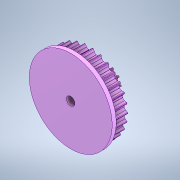
# Autodesk Inventor part: TransmissionCenterBigPulley HTD3M
Saved by Autodesk Inventor 2022.2 (Build 262287000, 287)
## iProperties
CustomPartVersion: 1
Created: 2022-01-04
Part Number: TransmissionCenterBigPulley HTD3M
Material: Steel
Document SubType Name: Modeling
Designer: Jochen
Density: 1 g/cm^3
Appearance: Steel
Author: Jochen
Autodesk Inventor part; units mm, degrees
ref_plane "YZ Plane" through (0, 0, 0) normal (1, 0, 0) x (0, 1, 0)
ref_plane "XZ Plane" through (0, 0, 0) normal (0, 1, 0) x (-1, 0, 0)
ref_plane "XY Plane" through (0, 0, 0) normal (0, 0, 1) x (1, 0, 0)
sketch "Pulley" plane through (0, 0, 0) normal (0, 0, 1) x (1, 0, 0)
  line L0 (0, -20.7693) -> (0, 20.7693) construction
  line L1 (-20.7693, 0) -> (20.7693, 0) construction
  circle A0 centre (0, 0) radius 14
  circle A1 centre (0, 0) radius 1.5
  arc A2 (-1.5293, 13.8609) -> (-1.6879, 13.7364) centre (-1.5084, 13.671) ccw
  arc A3 (-1.3859, 13.876) -> (-1.5293, 13.8609) centre (0, 0) ccw
  arc A4 (-1.205, 13.7871) -> (-1.3859, 13.876) centre (-1.3669, 13.6859) ccw
  line L2 (-1.205, 13.7871) -> (-0.8141, 13.1617)
  arc A5 (-0.8141, 13.1617) -> (-0.028, 12.726) centre (-0.028, 13.653) ccw
  line L3 (-0.028, 12.726) -> (0.028, 12.726)
  arc A6 (0.028, 12.726) -> (0.8141, 13.1617) centre (0.028, 13.653) ccw
  line L4 (0.8141, 13.1617) -> (1.205, 13.7871)
  arc A7 (1.3859, 13.876) -> (1.205, 13.7871) centre (1.3669, 13.6859) ccw
  arc A8 (1.5293, 13.8609) -> (1.3859, 13.876) centre (0, 0) ccw
  arc A9 (1.6879, 13.7364) -> (1.5293, 13.8609) centre (1.5084, 13.671) ccw
  line L5 (1.6879, 13.7364) -> (1.9402, 13.0434)
  arc A10 (1.9402, 13.0434) -> (2.6185, 12.4537) centre (2.8112, 13.3605) ccw
  line L6 (2.6185, 12.4537) -> (2.6733, 12.4421)
  arc A11 (2.6733, 12.4421) -> (3.5328, 12.7048) centre (2.866, 13.3488) ccw
  line L7 (3.5328, 12.7048) -> (4.0451, 13.2353)
  arc A12 (4.2406, 13.2846) -> (4.0451, 13.2353) centre (4.1825, 13.1026) ccw
  arc A13 (4.3778, 13.24) -> (4.2406, 13.2846) centre (0, 0) ccw
  arc A14 (4.5069, 13.0853) -> (4.3778, 13.24) centre (4.3178, 13.0587) ccw
  line L8 (4.5069, 13.0853) -> (4.6096, 12.3549)
  arc A15 (4.6096, 12.3549) -> (5.1506, 11.6372) centre (5.5276, 12.484) ccw
  line L9 (5.1506, 11.6372) -> (5.2017, 11.6144)
  arc A16 (5.2017, 11.6144) -> (6.0971, 11.6927) centre (5.5788, 12.4612) ccw
  line L10 (6.0971, 11.6927) -> (6.7085, 12.1051)
  arc A17 (6.91, 12.1126) -> (6.7085, 12.1051) centre (6.8153, 11.9467) ccw
  arc A18 (7.0348, 12.0405) -> (6.91, 12.1126) centre (0, 0) ccw
  arc A19 (7.129, 11.8623) -> (7.0348, 12.0405) centre (6.9385, 11.8756) ccw
  line L11 (7.129, 11.8623) -> (7.0776, 11.1266)
  arc A20 (7.0776, 11.1266) -> (7.4575, 10.312) centre (8.0024, 11.062) ccw
  line L12 (7.4575, 10.312) -> (7.5028, 10.2791)
  arc A21 (7.5028, 10.2791) -> (8.3949, 10.1695) centre (8.0477, 11.0291) ccw
  line L13 (8.3949, 10.1695) -> (9.0787, 10.4458)
  arc A22 (9.2773, 10.4113) -> (9.0787, 10.4458) centre (9.1503, 10.2687) ccw
  arc A23 (9.3845, 10.3148) -> (9.2773, 10.4113) centre (0, 0) ccw
  arc A24 (9.4395, 10.1209) -> (9.3845, 10.3148) centre (9.2559, 10.1735) ccw
  line L14 (9.4395, 10.1209) -> (9.2363, 9.4119)
  arc A25 (9.2363, 9.4119) -> (9.4385, 8.5362) centre (10.1274, 9.1564) ccw
  line L15 (9.4385, 8.5362) -> (9.476, 8.4945)
  arc A26 (9.476, 8.4945) -> (10.3258, 8.2019) centre (10.1649, 9.1148) ccw
  line L16 (10.3258, 8.2019) -> (11.0521, 8.3299)
  arc A27 (11.2392, 8.2549) -> (11.0521, 8.3299) centre (11.0853, 8.1418) ccw
  arc A28 (11.324, 8.1382) -> (11.2392, 8.2549) centre (0, 0) ccw
  arc A29 (11.3375, 7.9371) -> (11.324, 8.1382) centre (11.1689, 8.0268) ccw
  line L17 (11.3375, 7.9371) -> (10.9913, 7.2859)
  arc A30 (10.9913, 7.2859) -> (11.007, 6.3872) centre (11.8098, 6.8507) ccw
  line L18 (11.007, 6.3872) -> (11.035, 6.3388)
  arc A31 (11.035, 6.3388) -> (11.8054, 5.8758) centre (11.8378, 6.8023) ccw
  line L19 (11.8054, 5.8758) -> (12.5425, 5.85)
  arc A32 (12.7099, 5.7377) -> (12.5425, 5.85) centre (12.5358, 5.6591) ccw
  arc A33 (12.7685, 5.606) -> (12.7099, 5.7377) centre (0, 0) ccw
  arc A34 (12.74, 5.4065) -> (12.7685, 5.606) centre (12.5937, 5.5292) ccw
  line L20 (12.74, 5.4065) -> (12.266, 4.8415)
  arc A35 (12.266, 4.8415) -> (12.0945, 3.9592) centre (12.9761, 4.2456) ccw
  line L21 (12.0945, 3.9592) -> (12.1118, 3.9059)
  arc A36 (12.1118, 3.9059) -> (12.7691, 3.2929) centre (12.9934, 4.1924) ccw
  line L22 (12.7691, 3.2929) -> (13.4847, 3.1145)
  arc A37 (13.6251, 2.9698) -> (13.4847, 3.1145) centre (13.4385, 2.9291) ccw
  arc A38 (13.6551, 2.8288) -> (13.6251, 2.9698) centre (0, 0) ccw
  arc A39 (13.5856, 2.6395) -> (13.6551, 2.8288) centre (13.468, 2.79) ccw
  line L23 (13.5856, 2.6395) -> (13.0045, 2.1854)
  arc A40 (13.0045, 2.1854) -> (12.6534, 1.3581) centre (13.5753, 1.455) ccw
  line L24 (12.6534, 1.3581) -> (12.6592, 1.3024)
  arc A41 (12.6592, 1.3024) -> (13.1747, 0.5661) centre (13.5811, 1.3993) ccw
  line L25 (13.1747, 0.5661) -> (13.8376, 0.2428)
  arc A42 (13.9448, 0.0721) -> (13.8376, 0.2428) centre (13.7538, 0.0711) ccw
  arc A43 (13.9448, -0.0721) -> (13.9448, 0.0721) centre (0, 0) ccw
  arc A44 (13.8376, -0.2428) -> (13.9448, -0.0721) centre (13.7538, -0.0711) ccw
  line L26 (13.8376, -0.2428) -> (13.1747, -0.5661)
  arc A45 (13.1747, -0.5661) -> (12.6592, -1.3024) centre (13.5811, -1.3993) ccw
  line L27 (12.6592, -1.3024) -> (12.6534, -1.3581)
  arc A46 (12.6534, -1.3581) -> (13.0045, -2.1854) centre (13.5753, -1.455) ccw
  line L28 (13.0045, -2.1854) -> (13.5856, -2.6395)
  arc A47 (13.6551, -2.8288) -> (13.5856, -2.6395) centre (13.468, -2.79) ccw
  arc A48 (13.6251, -2.9698) -> (13.6551, -2.8288) centre (0, 0) ccw
  arc A49 (13.4847, -3.1145) -> (13.6251, -2.9698) centre (13.4385, -2.9291) ccw
  line L29 (13.4847, -3.1145) -> (12.7691, -3.2929)
  arc A50 (12.7691, -3.2929) -> (12.1118, -3.9059) centre (12.9934, -4.1924) ccw
  line L30 (12.1118, -3.9059) -> (12.0945, -3.9592)
  arc A51 (12.0945, -3.9592) -> (12.266, -4.8415) centre (12.9761, -4.2456) ccw
  line L31 (12.266, -4.8415) -> (12.74, -5.4065)
  arc A52 (12.7685, -5.606) -> (12.74, -5.4065) centre (12.5937, -5.5292) ccw
  arc A53 (12.7099, -5.7377) -> (12.7685, -5.606) centre (0, 0) ccw
  arc A54 (12.5425, -5.85) -> (12.7099, -5.7377) centre (12.5358, -5.6591) ccw
  line L32 (12.5425, -5.85) -> (11.8054, -5.8758)
  arc A55 (11.8054, -5.8758) -> (11.035, -6.3388) centre (11.8378, -6.8023) ccw
  line L33 (11.035, -6.3388) -> (11.007, -6.3872)
  arc A56 (11.007, -6.3872) -> (10.9913, -7.2859) centre (11.8098, -6.8507) ccw
  line L34 (10.9913, -7.2859) -> (11.3375, -7.9371)
  arc A57 (11.324, -8.1382) -> (11.3375, -7.9371) centre (11.1689, -8.0268) ccw
  arc A58 (11.2392, -8.2549) -> (11.324, -8.1382) centre (0, 0) ccw
  arc A59 (11.0521, -8.3299) -> (11.2392, -8.2549) centre (11.0853, -8.1418) ccw
  line L35 (11.0521, -8.3299) -> (10.3258, -8.2019)
  arc A60 (10.3258, -8.2019) -> (9.476, -8.4945) centre (10.1649, -9.1148) ccw
  line L36 (9.476, -8.4945) -> (9.4385, -8.5362)
  arc A61 (9.4385, -8.5362) -> (9.2363, -9.4119) centre (10.1274, -9.1564) ccw
  line L37 (9.2363, -9.4119) -> (9.4395, -10.1209)
  arc A62 (9.3845, -10.3148) -> (9.4395, -10.1209) centre (9.2559, -10.1735) ccw
  arc A63 (9.2773, -10.4113) -> (9.3845, -10.3148) centre (0, 0) ccw
  arc A64 (9.0787, -10.4458) -> (9.2773, -10.4113) centre (9.1503, -10.2687) ccw
  line L38 (9.0787, -10.4458) -> (8.3949, -10.1695)
  arc A65 (8.3949, -10.1695) -> (7.5028, -10.2791) centre (8.0477, -11.0291) ccw
  line L39 (7.5028, -10.2791) -> (7.4575, -10.312)
  arc A66 (7.4575, -10.312) -> (7.0776, -11.1266) centre (8.0024, -11.062) ccw
  line L40 (7.0776, -11.1266) -> (7.129, -11.8623)
  arc A67 (7.0348, -12.0405) -> (7.129, -11.8623) centre (6.9385, -11.8756) ccw
  arc A68 (6.91, -12.1126) -> (7.0348, -12.0405) centre (0, 0) ccw
  arc A69 (6.7085, -12.1051) -> (6.91, -12.1126) centre (6.8153, -11.9467) ccw
  line L41 (6.7085, -12.1051) -> (6.0971, -11.6927)
  arc A70 (6.0971, -11.6927) -> (5.2017, -11.6144) centre (5.5788, -12.4612) ccw
  line L42 (5.2017, -11.6144) -> (5.1506, -11.6372)
  arc A71 (5.1506, -11.6372) -> (4.6096, -12.3549) centre (5.5276, -12.484) ccw
  line L43 (4.6096, -12.3549) -> (4.5069, -13.0853)
  arc A72 (4.3778, -13.24) -> (4.5069, -13.0853) centre (4.3178, -13.0587) ccw
  arc A73 (4.2406, -13.2846) -> (4.3778, -13.24) centre (0, 0) ccw
  arc A74 (4.0451, -13.2353) -> (4.2406, -13.2846) centre (4.1825, -13.1026) ccw
  line L44 (4.0451, -13.2353) -> (3.5328, -12.7048)
  arc A75 (3.5328, -12.7048) -> (2.6733, -12.4421) centre (2.866, -13.3488) ccw
  line L45 (2.6733, -12.4421) -> (2.6185, -12.4537)
  arc A76 (2.6185, -12.4537) -> (1.9402, -13.0434) centre (2.8112, -13.3605) ccw
  line L46 (1.9402, -13.0434) -> (1.6879, -13.7364)
  arc A77 (1.5293, -13.8609) -> (1.6879, -13.7364) centre (1.5084, -13.671) ccw
  arc A78 (1.3859, -13.876) -> (1.5293, -13.8609) centre (0, 0) ccw
  arc A79 (1.205, -13.7871) -> (1.3859, -13.876) centre (1.3669, -13.6859) ccw
  line L47 (1.205, -13.7871) -> (0.8141, -13.1617)
  arc A80 (0.8141, -13.1617) -> (0.028, -12.726) centre (0.028, -13.653) ccw
  line L48 (0.028, -12.726) -> (-0.028, -12.726)
  arc A81 (-0.028, -12.726) -> (-0.8141, -13.1617) centre (-0.028, -13.653) ccw
  line L49 (-0.8141, -13.1617) -> (-1.205, -13.7871)
  arc A82 (-1.3859, -13.876) -> (-1.205, -13.7871) centre (-1.3669, -13.6859) ccw
  arc A83 (-1.5293, -13.8609) -> (-1.3859, -13.876) centre (0, 0) ccw
  arc A84 (-1.6879, -13.7364) -> (-1.5293, -13.8609) centre (-1.5084, -13.671) ccw
  line L50 (-1.6879, -13.7364) -> (-1.9402, -13.0434)
  arc A85 (-1.9402, -13.0434) -> (-2.6185, -12.4537) centre (-2.8112, -13.3605) ccw
  line L51 (-2.6185, -12.4537) -> (-2.6733, -12.4421)
  arc A86 (-2.6733, -12.4421) -> (-3.5328, -12.7048) centre (-2.866, -13.3488) ccw
  line L52 (-3.5328, -12.7048) -> (-4.0451, -13.2353)
  arc A87 (-4.2406, -13.2846) -> (-4.0451, -13.2353) centre (-4.1825, -13.1026) ccw
  arc A88 (-4.3778, -13.24) -> (-4.2406, -13.2846) centre (0, 0) ccw
  arc A89 (-4.5069, -13.0853) -> (-4.3778, -13.24) centre (-4.3178, -13.0587) ccw
  line L53 (-4.5069, -13.0853) -> (-4.6096, -12.3549)
  arc A90 (-4.6096, -12.3549) -> (-5.1506, -11.6372) centre (-5.5276, -12.484) ccw
  line L54 (-5.1506, -11.6372) -> (-5.2017, -11.6144)
  arc A91 (-5.2017, -11.6144) -> (-6.0971, -11.6927) centre (-5.5788, -12.4612) ccw
  line L55 (-6.0971, -11.6927) -> (-6.7085, -12.1051)
  arc A92 (-6.91, -12.1126) -> (-6.7085, -12.1051) centre (-6.8153, -11.9467) ccw
  arc A93 (-7.0348, -12.0405) -> (-6.91, -12.1126) centre (0, 0) ccw
  arc A94 (-7.129, -11.8623) -> (-7.0348, -12.0405) centre (-6.9385, -11.8756) ccw
  line L56 (-7.129, -11.8623) -> (-7.0776, -11.1266)
  arc A95 (-7.0776, -11.1266) -> (-7.4575, -10.312) centre (-8.0024, -11.062) ccw
  line L57 (-7.4575, -10.312) -> (-7.5028, -10.2791)
  arc A96 (-7.5028, -10.2791) -> (-8.3949, -10.1695) centre (-8.0477, -11.0291) ccw
  line L58 (-8.3949, -10.1695) -> (-9.0787, -10.4458)
  arc A97 (-9.2773, -10.4113) -> (-9.0787, -10.4458) centre (-9.1503, -10.2687) ccw
  arc A98 (-9.3845, -10.3148) -> (-9.2773, -10.4113) centre (0, 0) ccw
  arc A99 (-9.4395, -10.1209) -> (-9.3845, -10.3148) centre (-9.2559, -10.1735) ccw
  line L59 (-9.4395, -10.1209) -> (-9.2363, -9.4119)
  arc A100 (-9.2363, -9.4119) -> (-9.4385, -8.5362) centre (-10.1274, -9.1564) ccw
  line L60 (-9.4385, -8.5362) -> (-9.476, -8.4945)
  arc A101 (-9.476, -8.4945) -> (-10.3258, -8.2019) centre (-10.1649, -9.1148) ccw
  line L61 (-10.3258, -8.2019) -> (-11.0521, -8.3299)
  arc A102 (-11.2392, -8.2549) -> (-11.0521, -8.3299) centre (-11.0853, -8.1418) ccw
  arc A103 (-11.324, -8.1382) -> (-11.2392, -8.2549) centre (0, 0) ccw
  arc A104 (-11.3375, -7.9371) -> (-11.324, -8.1382) centre (-11.1689, -8.0268) ccw
  line L62 (-11.3375, -7.9371) -> (-10.9913, -7.2859)
  arc A105 (-10.9913, -7.2859) -> (-11.007, -6.3872) centre (-11.8098, -6.8507) ccw
  line L63 (-11.007, -6.3872) -> (-11.035, -6.3388)
  arc A106 (-11.035, -6.3388) -> (-11.8054, -5.8758) centre (-11.8378, -6.8023) ccw
  line L64 (-11.8054, -5.8758) -> (-12.5425, -5.85)
  arc A107 (-12.7099, -5.7377) -> (-12.5425, -5.85) centre (-12.5358, -5.6591) ccw
  arc A108 (-12.7685, -5.606) -> (-12.7099, -5.7377) centre (0, 0) ccw
  arc A109 (-12.74, -5.4065) -> (-12.7685, -5.606) centre (-12.5937, -5.5292) ccw
  line L65 (-12.74, -5.4065) -> (-12.266, -4.8415)
  arc A110 (-12.266, -4.8415) -> (-12.0945, -3.9592) centre (-12.9761, -4.2456) ccw
  line L66 (-12.0945, -3.9592) -> (-12.1118, -3.9059)
  arc A111 (-12.1118, -3.9059) -> (-12.7691, -3.2929) centre (-12.9934, -4.1924) ccw
  line L67 (-12.7691, -3.2929) -> (-13.4847, -3.1145)
  arc A112 (-13.6251, -2.9698) -> (-13.4847, -3.1145) centre (-13.4385, -2.9291) ccw
  arc A113 (-13.6551, -2.8288) -> (-13.6251, -2.9698) centre (0, 0) ccw
  arc A114 (-13.5856, -2.6395) -> (-13.6551, -2.8288) centre (-13.468, -2.79) ccw
  line L68 (-13.5856, -2.6395) -> (-13.0045, -2.1854)
  arc A115 (-13.0045, -2.1854) -> (-12.6534, -1.3581) centre (-13.5753, -1.455) ccw
  line L69 (-12.6534, -1.3581) -> (-12.6592, -1.3024)
  arc A116 (-12.6592, -1.3024) -> (-13.1747, -0.5661) centre (-13.5811, -1.3993) ccw
  line L70 (-13.1747, -0.5661) -> (-13.8376, -0.2428)
  arc A117 (-13.9448, -0.0721) -> (-13.8376, -0.2428) centre (-13.7538, -0.0711) ccw
  arc A118 (-13.9448, 0.0721) -> (-13.9448, -0.0721) centre (0, 0) ccw
  arc A119 (-13.8376, 0.2428) -> (-13.9448, 0.0721) centre (-13.7538, 0.0711) ccw
  line L71 (-13.8376, 0.2428) -> (-13.1747, 0.5661)
  arc A120 (-13.1747, 0.5661) -> (-12.6592, 1.3024) centre (-13.5811, 1.3993) ccw
  line L72 (-12.6592, 1.3024) -> (-12.6534, 1.3581)
  arc A121 (-12.6534, 1.3581) -> (-13.0045, 2.1854) centre (-13.5753, 1.455) ccw
  line L73 (-13.0045, 2.1854) -> (-13.5856, 2.6395)
  arc A122 (-13.6551, 2.8288) -> (-13.5856, 2.6395) centre (-13.468, 2.79) ccw
  arc A123 (-13.6251, 2.9698) -> (-13.6551, 2.8288) centre (0, 0) ccw
  arc A124 (-13.4847, 3.1145) -> (-13.6251, 2.9698) centre (-13.4385, 2.9291) ccw
  line L74 (-13.4847, 3.1145) -> (-12.7691, 3.2929)
  arc A125 (-12.7691, 3.2929) -> (-12.1118, 3.9059) centre (-12.9934, 4.1924) ccw
  line L75 (-12.1118, 3.9059) -> (-12.0945, 3.9592)
  arc A126 (-12.0945, 3.9592) -> (-12.266, 4.8415) centre (-12.9761, 4.2456) ccw
  line L76 (-12.266, 4.8415) -> (-12.74, 5.4065)
  arc A127 (-12.7685, 5.606) -> (-12.74, 5.4065) centre (-12.5937, 5.5292) ccw
  arc A128 (-12.7099, 5.7377) -> (-12.7685, 5.606) centre (0, 0) ccw
  arc A129 (-12.5425, 5.85) -> (-12.7099, 5.7377) centre (-12.5358, 5.6591) ccw
  line L77 (-12.5425, 5.85) -> (-11.8054, 5.8758)
  arc A130 (-11.8054, 5.8758) -> (-11.035, 6.3388) centre (-11.8378, 6.8023) ccw
  line L78 (-11.035, 6.3388) -> (-11.007, 6.3872)
  arc A131 (-11.007, 6.3872) -> (-10.9913, 7.2859) centre (-11.8098, 6.8507) ccw
  line L79 (-10.9913, 7.2859) -> (-11.3375, 7.9371)
  arc A132 (-11.324, 8.1382) -> (-11.3375, 7.9371) centre (-11.1689, 8.0268) ccw
  arc A133 (-11.2392, 8.2549) -> (-11.324, 8.1382) centre (0, 0) ccw
  arc A134 (-11.0521, 8.3299) -> (-11.2392, 8.2549) centre (-11.0853, 8.1418) ccw
  line L80 (-11.0521, 8.3299) -> (-10.3258, 8.2019)
  arc A135 (-10.3258, 8.2019) -> (-9.476, 8.4945) centre (-10.1649, 9.1148) ccw
  line L81 (-9.476, 8.4945) -> (-9.4385, 8.5362)
  arc A136 (-9.4385, 8.5362) -> (-9.2363, 9.4119) centre (-10.1274, 9.1564) ccw
  line L82 (-9.2363, 9.4119) -> (-9.4395, 10.1209)
  arc A137 (-9.3845, 10.3148) -> (-9.4395, 10.1209) centre (-9.2559, 10.1735) ccw
  arc A138 (-9.2773, 10.4113) -> (-9.3845, 10.3148) centre (0, 0) ccw
  arc A139 (-9.0787, 10.4458) -> (-9.2773, 10.4113) centre (-9.1503, 10.2687) ccw
  line L83 (-9.0787, 10.4458) -> (-8.3949, 10.1695)
  arc A140 (-8.3949, 10.1695) -> (-7.5028, 10.2791) centre (-8.0477, 11.0291) ccw
  line L84 (-7.5028, 10.2791) -> (-7.4575, 10.312)
  arc A141 (-7.4575, 10.312) -> (-7.0776, 11.1266) centre (-8.0024, 11.062) ccw
  line L85 (-7.0776, 11.1266) -> (-7.129, 11.8623)
  arc A142 (-7.0348, 12.0405) -> (-7.129, 11.8623) centre (-6.9385, 11.8756) ccw
  arc A143 (-6.91, 12.1126) -> (-7.0348, 12.0405) centre (0, 0) ccw
  arc A144 (-6.7085, 12.1051) -> (-6.91, 12.1126) centre (-6.8153, 11.9467) ccw
  line L86 (-6.7085, 12.1051) -> (-6.0971, 11.6927)
  arc A145 (-6.0971, 11.6927) -> (-5.2017, 11.6144) centre (-5.5788, 12.4612) ccw
  line L87 (-5.2017, 11.6144) -> (-5.1506, 11.6372)
  arc A146 (-5.1506, 11.6372) -> (-4.6096, 12.3549) centre (-5.5276, 12.484) ccw
  line L88 (-4.6096, 12.3549) -> (-4.5069, 13.0853)
  arc A147 (-4.3778, 13.24) -> (-4.5069, 13.0853) centre (-4.3178, 13.0587) ccw
  arc A148 (-4.2406, 13.2846) -> (-4.3778, 13.24) centre (0, 0) ccw
  arc A149 (-4.0451, 13.2353) -> (-4.2406, 13.2846) centre (-4.1825, 13.1026) ccw
  line L89 (-4.0451, 13.2353) -> (-3.5328, 12.7048)
  arc A150 (-3.5328, 12.7048) -> (-2.6733, 12.4421) centre (-2.866, 13.3488) ccw
  line L90 (-2.6733, 12.4421) -> (-2.6185, 12.4537)
  arc A151 (-2.6185, 12.4537) -> (-1.9402, 13.0434) centre (-2.8112, 13.3605) ccw
  line L91 (-1.9402, 13.0434) -> (-1.6879, 13.7364)
  circle A152 centre (0, 0) radius 14.3352
  circle A153 centre (0, 0) radius 14.8352
  dimension "d56" = 3
  dimension "d63" = 28.6705
  dimension "d64" = 0.5
  constraints: 300 point on circle, 180 end point, 154 centre point, 2 coincident
  measures "d56" diameter of A1
  measures "d63" diameter of A152
  measures "d64" radial gap between concentric circles of A153 A152
extrude "Extrusion11" add sketch "Pulley" along normal mid plane 4.75 contours A3 A4 L2 A5 L3 A6 L4 A7 A8 A9 L5 A10 L6 A11 L7 A12 A13 A14 L8 A15 L9 A16 L10 A17 A18 A19 L11 A20 L12 A21 L13 A22 A23 A24 L14 A25 L15 A26 L16 A27 A28 A29 L17 A30 L18 A31 L19 A32 A33 A34 L20 A35 L21 A36 L22 A37 A38 A39 L23 A40 L24 A41 L25 A42 A43 A44 L26 A45 L27 A46 L28 A47 A48 A49 L29 A50 L30 A51 L31 A52 A53 A54 L32 A55 L33 A56 L34 A57 A58 A59 L35 A60 L36 A61 L37 A62 A63 A64 L38 A65 L39 A66 L40 A67 A68 A69 L41 A70 L42 A71 L43 A72 A73 A74 L44 A75 L45 A76 L46 A77 A78 A79 L47 A80 L48 A81 L49 A82 A83 A84 L50 A85 L51 A86 L52 A87 A88 A89 L53 A90 L54 A91 L55 A92 A93 A94 L56 A95 L57 A96 L58 A97 A98 A99 L59 A100 L60 A101 L61 A102 A103 A104 L62 A105 L63 A106 L64 A107 A108 A109 L65 A110 L66 A111 L67 A112 A113 A114 L68 A115 L69 A116 L70 A117 A118 A119 L71 A120 L72 A121 L73 A122 A123 A124 L74 A125 L75 A126 L76 A127 A128 A129 L77 A130 L78 A131 L79 A132 A133 A134 L80 A135 L81 A136 L82 A137 A138 A139 L83 A140 L84 A141 L85 A142 A143 A144 L86 A145 L87 A146 L88 A147 A148 A149 L89 A150 L90 A151 L91 A2
extrude "Extrusion12" add sketch "Pulley" along normal blind 1.75 from surface at 2.375 contours A0 | A3 A4 L2 A5 L3 A6 L4 A7 A8 A9 L5 A10 L6 A11 L7 A12 A13 A14 L8 A15 L9 A16 L10 A17 A18 A19 L11 A20 L12 A21 L13 A22 A23 A24 L14 A25 L15 A26 L16 A27 A28 A29 L17 A30 L18 A31 L19 A32 A33 A34 L20 A35 L21 A36 L22 A37 A38 A39 L23 A40 L24 A41 L25 A42 A43 A44 L26 A45 L27 A46 L28 A47 A48 A49 L29 A50 L30 A51 L31 A52 A53 A54 L32 A55 L33 A56 L34 A57 A58 A59 L35 A60 L36 A61 L37 A62 A63 A64 L38 A65 L39 A66 L40 A67 A68 A69 L41 A70 L42 A71 L43 A72 A73 A74 L44 A75 L45 A76 L46 A77 A78 A79 L47 A80 L48 A81 L49 A82 A83 A84 L50 A85 L51 A86 L52 A87 A88 A89 L53 A90 L54 A91 L55 A92 A93 A94 L56 A95 L57 A96 L58 A97 A98 A99 L59 A100 L60 A101 L61 A102 A103 A104 L62 A105 L63 A106 L64 A107 A108 A109 L65 A110 L66 A111 L67 A112 A113 A114 L68 A115 L69 A116 L70 A117 A118 A119 L71 A120 L72 A121 L73 A122 A123 A124 L74 A125 L75 A126 L76 A127 A128 A129 L77 A130 L78 A131 L79 A132 A133 A134 L80 A135 L81 A136 L82 A137 A138 A139 L83 A140 L84 A141 L85 A142 A143 A144 L86 A145 L87 A146 L88 A147 A148 A149 L89 A150 L90 A151 L91 A2 | A152 | A153
chamfer "Chamfer4" distance 0.8 distance2 0.3 1 edges at (-14.8352, 0, 2.375) measured on face at (0.4104, 14.4248, 2.375)
sketch "Sketch9" plane through (0, 0, -2.375) normal (0, 0, -1) x (-1, 0, 0)
  circle A0 centre (0, 0) radius 5
  line L0 (0.8939, 3.7122) -> (1.1141, 4.1058)
  arc A1 (1.3267, 4.19) -> (1.1141, 4.1058) centre (1.272, 4.0174) ccw
  arc A2 (1.3895, 4.1696) -> (1.3267, 4.19) centre (0, 0) ccw
  arc A3 (1.512, 3.9765) -> (1.3895, 4.1696) centre (1.3323, 3.9979) ccw
  line L1 (1.512, 3.9765) -> (1.4588, 3.5286)
  arc A4 (1.4588, 3.5286) -> (1.8604, 2.6099) centre (2.4429, 3.4117) ccw
  line L2 (1.8604, 2.6099) -> (1.9073, 2.5759)
  arc A5 (1.9073, 2.5759) -> (2.9051, 2.4778) centre (2.4898, 3.3776) ccw
  line L3 (2.9051, 2.4778) -> (3.3146, 2.6668)
  arc A6 (3.5361, 2.61) -> (3.3146, 2.6668) centre (3.3905, 2.5025) ccw
  arc A7 (3.5749, 2.5565) -> (3.5361, 2.61) centre (0, 0) ccw
  arc A8 (3.5606, 2.3283) -> (3.5749, 2.5565) centre (3.4277, 2.4512) ccw
  line L4 (3.5606, 2.3283) -> (3.2543, 1.9972)
  arc A9 (3.2543, 1.9972) -> (3.0392, 1.018) centre (3.9817, 1.3242) ccw
  line L5 (3.0392, 1.018) -> (3.0571, 0.9628)
  arc A10 (3.0571, 0.9628) -> (3.8067, 0.297) centre (3.9996, 1.2691) ccw
  line L6 (3.8067, 0.297) -> (4.2491, 0.2092)
  arc A11 (4.3949, 0.033) -> (4.2491, 0.2092) centre (4.2139, 0.0317) ccw
  arc A12 (4.3949, -0.033) -> (4.3949, 0.033) centre (0, 0) ccw
  arc A13 (4.2491, -0.2092) -> (4.3949, -0.033) centre (4.2139, -0.0317) ccw
  line L7 (4.2491, -0.2092) -> (3.8067, -0.297)
  arc A14 (3.8067, -0.297) -> (3.0571, -0.9628) centre (3.9996, -1.2691) ccw
  line L8 (3.0571, -0.9628) -> (3.0392, -1.018)
  arc A15 (3.0392, -1.018) -> (3.2543, -1.9972) centre (3.9817, -1.3242) ccw
  line L9 (3.2543, -1.9972) -> (3.5606, -2.3283)
  arc A16 (3.5749, -2.5565) -> (3.5606, -2.3283) centre (3.4277, -2.4512) ccw
  arc A17 (3.5361, -2.61) -> (3.5749, -2.5565) centre (0, 0) ccw
  arc A18 (3.3146, -2.6668) -> (3.5361, -2.61) centre (3.3905, -2.5025) ccw
  line L10 (3.3146, -2.6668) -> (2.9051, -2.4778)
  arc A19 (2.9051, -2.4778) -> (1.9073, -2.5759) centre (2.4898, -3.3776) ccw
  line L11 (1.9073, -2.5759) -> (1.8604, -2.6099)
  arc A20 (1.8604, -2.6099) -> (1.4588, -3.5286) centre (2.4429, -3.4117) ccw
  line L12 (1.4588, -3.5286) -> (1.512, -3.9765)
  arc A21 (1.3895, -4.1696) -> (1.512, -3.9765) centre (1.3323, -3.9979) ccw
  arc A22 (1.3267, -4.19) -> (1.3895, -4.1696) centre (0, 0) ccw
  arc A23 (1.1141, -4.1058) -> (1.3267, -4.19) centre (1.272, -4.0174) ccw
  line L13 (1.1141, -4.1058) -> (0.8939, -3.7122)
  arc A24 (0.8939, -3.7122) -> (0.029, -3.205) centre (0.029, -4.196) ccw
  line L14 (0.029, -3.205) -> (-0.029, -3.205)
  arc A25 (-0.029, -3.205) -> (-0.8939, -3.7122) centre (-0.029, -4.196) ccw
  line L15 (-0.8939, -3.7122) -> (-1.1141, -4.1058)
  arc A26 (-1.3267, -4.19) -> (-1.1141, -4.1058) centre (-1.272, -4.0174) ccw
  arc A27 (-1.3895, -4.1696) -> (-1.3267, -4.19) centre (0, 0) ccw
  arc A28 (-1.512, -3.9765) -> (-1.3895, -4.1696) centre (-1.3323, -3.9979) ccw
  line L16 (-1.512, -3.9765) -> (-1.4588, -3.5286)
  arc A29 (-1.4588, -3.5286) -> (-1.8604, -2.6099) centre (-2.4429, -3.4117) ccw
  line L17 (-1.8604, -2.6099) -> (-1.9073, -2.5759)
  arc A30 (-1.9073, -2.5759) -> (-2.9051, -2.4778) centre (-2.4898, -3.3776) ccw
  line L18 (-2.9051, -2.4778) -> (-3.3146, -2.6668)
  arc A31 (-3.5361, -2.61) -> (-3.3146, -2.6668) centre (-3.3905, -2.5025) ccw
  arc A32 (-3.5749, -2.5565) -> (-3.5361, -2.61) centre (0, 0) ccw
  arc A33 (-3.5606, -2.3283) -> (-3.5749, -2.5565) centre (-3.4277, -2.4512) ccw
  line L19 (-3.5606, -2.3283) -> (-3.2543, -1.9972)
  arc A34 (-3.2543, -1.9972) -> (-3.0392, -1.018) centre (-3.9817, -1.3242) ccw
  line L20 (-3.0392, -1.018) -> (-3.0571, -0.9628)
  arc A35 (-3.0571, -0.9628) -> (-3.8067, -0.297) centre (-3.9996, -1.2691) ccw
  line L21 (-3.8067, -0.297) -> (-4.2491, -0.2092)
  arc A36 (-4.3949, -0.033) -> (-4.2491, -0.2092) centre (-4.2139, -0.0317) ccw
  arc A37 (-4.3949, 0.033) -> (-4.3949, -0.033) centre (0, 0) ccw
  arc A38 (-4.2491, 0.2092) -> (-4.3949, 0.033) centre (-4.2139, 0.0317) ccw
  line L22 (-4.2491, 0.2092) -> (-3.8067, 0.297)
  arc A39 (-3.8067, 0.297) -> (-3.0571, 0.9628) centre (-3.9996, 1.2691) ccw
  line L23 (-3.0571, 0.9628) -> (-3.0392, 1.018)
  arc A40 (-3.0392, 1.018) -> (-3.2543, 1.9972) centre (-3.9817, 1.3242) ccw
  line L24 (-3.2543, 1.9972) -> (-3.5606, 2.3283)
  arc A41 (-3.5749, 2.5565) -> (-3.5606, 2.3283) centre (-3.4277, 2.4512) ccw
  arc A42 (-3.5361, 2.61) -> (-3.5749, 2.5565) centre (0, 0) ccw
  arc A43 (-3.3146, 2.6668) -> (-3.5361, 2.61) centre (-3.3905, 2.5025) ccw
  line L25 (-3.3146, 2.6668) -> (-2.9051, 2.4778)
  arc A44 (-2.9051, 2.4778) -> (-1.9073, 2.5759) centre (-2.4898, 3.3776) ccw
  line L26 (-1.9073, 2.5759) -> (-1.8604, 2.6099)
  arc A45 (-1.8604, 2.6099) -> (-1.4588, 3.5286) centre (-2.4429, 3.4117) ccw
  line L27 (-1.4588, 3.5286) -> (-1.512, 3.9765)
  arc A46 (-1.3895, 4.1696) -> (-1.512, 3.9765) centre (-1.3323, 3.9979) ccw
  arc A47 (-1.3267, 4.19) -> (-1.3895, 4.1696) centre (0, 0) ccw
  arc A48 (-1.1141, 4.1058) -> (-1.3267, 4.19) centre (-1.272, 4.0174) ccw
  line L28 (-1.1141, 4.1058) -> (-0.8939, 3.7122)
  arc A49 (-0.8939, 3.7122) -> (-0.029, 3.205) centre (-0.029, 4.196) ccw
  line L29 (-0.029, 3.205) -> (0.029, 3.205)
  arc A50 (0.029, 3.205) -> (0.8939, 3.7122) centre (0.029, 4.196) ccw
  circle A51 centre (0, 0) radius 6.5
  circle A52 centre (0, 0) radius 5.1866
  arc A53 (-0.029, -3.405) -> (-0.7193, -3.8098) centre (-0.029, -4.196) ccw
  line L30 (-0.029, -3.405) -> (0.029, -3.405)
  arc A54 (0.7193, -3.8098) -> (0.029, -3.405) centre (0.029, -4.196) ccw
  line L31 (0.7193, -3.8098) -> (0.9395, -4.2034)
  arc A55 (0.9395, -4.2034) -> (1.387, -4.3807) centre (1.272, -4.0174) ccw
  arc A56 (1.387, -4.3807) -> (1.4527, -4.3593) centre (0, 0) ccw
  arc A57 (1.4527, -4.3593) -> (1.7106, -3.9529) centre (1.3323, -3.9979) ccw
  line L32 (1.7106, -3.9529) -> (1.6574, -3.505)
  arc A58 (1.9779, -2.7717) -> (1.6574, -3.505) centre (2.4429, -3.4117) ccw
  line L33 (1.9779, -2.7717) -> (2.0249, -2.7377)
  arc A59 (2.8213, -2.6594) -> (2.0249, -2.7377) centre (2.4898, -3.3776) ccw
  line L34 (2.8213, -2.6594) -> (3.2308, -2.8484)
  arc A60 (3.2308, -2.8484) -> (3.697, -2.7287) centre (3.3905, -2.5025) ccw
  arc A61 (3.697, -2.7287) -> (3.7376, -2.6729) centre (0, 0) ccw
  arc A62 (3.7376, -2.6729) -> (3.7074, -2.1925) centre (3.4277, -2.4512) ccw
  line L35 (3.7074, -2.1925) -> (3.4011, -1.8614)
  arc A63 (3.2294, -1.0798) -> (3.4011, -1.8614) centre (3.9817, -1.3242) ccw
  line L36 (3.2294, -1.0798) -> (3.2473, -1.0246)
  arc A64 (3.8456, -0.4932) -> (3.2473, -1.0246) centre (3.9996, -1.2691) ccw
  line L37 (3.8456, -0.4932) -> (4.288, -0.4054)
  arc A65 (4.288, -0.4054) -> (4.5949, -0.0345) centre (4.2139, -0.0317) ccw
  arc A66 (4.5949, -0.0345) -> (4.5949, 0.0345) centre (0, 0) ccw
  arc A67 (4.5949, 0.0345) -> (4.288, 0.4054) centre (4.2139, 0.0317) ccw
  line L38 (4.288, 0.4054) -> (3.8456, 0.4932)
  arc A68 (3.2473, 1.0246) -> (3.8456, 0.4932) centre (3.9996, 1.2691) ccw
  line L39 (3.2473, 1.0246) -> (3.2294, 1.0798)
  arc A69 (3.4011, 1.8614) -> (3.2294, 1.0798) centre (3.9817, 1.3242) ccw
  line L40 (3.4011, 1.8614) -> (3.7074, 2.1925)
  arc A70 (3.7074, 2.1925) -> (3.7376, 2.6729) centre (3.4277, 2.4512) ccw
  arc A71 (3.7376, 2.6729) -> (3.697, 2.7287) centre (0, 0) ccw
  arc A72 (3.697, 2.7287) -> (3.2308, 2.8484) centre (3.3905, 2.5025) ccw
  line L41 (3.2308, 2.8484) -> (2.8213, 2.6594)
  arc A73 (2.0249, 2.7377) -> (2.8213, 2.6594) centre (2.4898, 3.3776) ccw
  line L42 (2.0249, 2.7377) -> (1.9779, 2.7717)
  arc A74 (1.6574, 3.505) -> (1.9779, 2.7717) centre (2.4429, 3.4117) ccw
  line L43 (1.6574, 3.505) -> (1.7106, 3.9529)
  arc A75 (1.7106, 3.9529) -> (1.4527, 4.3593) centre (1.3323, 3.9979) ccw
  arc A76 (1.4527, 4.3593) -> (1.387, 4.3807) centre (0, 0) ccw
  arc A77 (1.387, 4.3807) -> (0.9395, 4.2034) centre (1.272, 4.0174) ccw
  line L44 (0.9395, 4.2034) -> (0.7193, 3.8098)
  arc A78 (0.029, 3.405) -> (0.7193, 3.8098) centre (0.029, 4.196) ccw
  line L45 (0.029, 3.405) -> (-0.029, 3.405)
  arc A79 (-0.7193, 3.8098) -> (-0.029, 3.405) centre (-0.029, 4.196) ccw
  line L46 (-0.7193, 3.8098) -> (-0.9395, 4.2034)
  arc A80 (-0.9395, 4.2034) -> (-1.387, 4.3807) centre (-1.272, 4.0174) ccw
  arc A81 (-1.387, 4.3807) -> (-1.4527, 4.3593) centre (0, 0) ccw
  arc A82 (-1.4527, 4.3593) -> (-1.7106, 3.9529) centre (-1.3323, 3.9979) ccw
  line L47 (-1.7106, 3.9529) -> (-1.6574, 3.505)
  arc A83 (-1.9779, 2.7717) -> (-1.6574, 3.505) centre (-2.4429, 3.4117) ccw
  line L48 (-1.9779, 2.7717) -> (-2.0249, 2.7377)
  arc A84 (-2.8213, 2.6594) -> (-2.0249, 2.7377) centre (-2.4898, 3.3776) ccw
  line L49 (-2.8213, 2.6594) -> (-3.2308, 2.8484)
  arc A85 (-3.2308, 2.8484) -> (-3.697, 2.7287) centre (-3.3905, 2.5025) ccw
  arc A86 (-3.697, 2.7287) -> (-3.7376, 2.6729) centre (0, 0) ccw
  arc A87 (-3.7376, 2.6729) -> (-3.7074, 2.1925) centre (-3.4277, 2.4512) ccw
  line L50 (-3.7074, 2.1925) -> (-3.4011, 1.8614)
  arc A88 (-3.2294, 1.0798) -> (-3.4011, 1.8614) centre (-3.9817, 1.3242) ccw
  line L51 (-3.2294, 1.0798) -> (-3.2473, 1.0246)
  arc A89 (-3.8456, 0.4932) -> (-3.2473, 1.0246) centre (-3.9996, 1.2691) ccw
  line L52 (-3.8456, 0.4932) -> (-4.288, 0.4054)
  arc A90 (-4.288, 0.4054) -> (-4.5949, 0.0345) centre (-4.2139, 0.0317) ccw
  arc A91 (-4.5949, 0.0345) -> (-4.5949, -0.0345) centre (0, 0) ccw
  arc A92 (-4.5949, -0.0345) -> (-4.288, -0.4054) centre (-4.2139, -0.0317) ccw
  line L53 (-4.288, -0.4054) -> (-3.8456, -0.4932)
  arc A93 (-3.2473, -1.0246) -> (-3.8456, -0.4932) centre (-3.9996, -1.2691) ccw
  line L54 (-3.2473, -1.0246) -> (-3.2294, -1.0798)
  arc A94 (-3.4011, -1.8614) -> (-3.2294, -1.0798) centre (-3.9817, -1.3242) ccw
  line L55 (-3.4011, -1.8614) -> (-3.7074, -2.1925)
  arc A95 (-3.7074, -2.1925) -> (-3.7376, -2.6729) centre (-3.4277, -2.4512) ccw
  arc A96 (-3.7376, -2.6729) -> (-3.697, -2.7287) centre (0, 0) ccw
  arc A97 (-3.697, -2.7287) -> (-3.2308, -2.8484) centre (-3.3905, -2.5025) ccw
  line L56 (-3.2308, -2.8484) -> (-2.8213, -2.6594)
  arc A98 (-2.0249, -2.7377) -> (-2.8213, -2.6594) centre (-2.4898, -3.3776) ccw
  line L57 (-2.0249, -2.7377) -> (-1.9779, -2.7717)
  arc A99 (-1.6574, -3.505) -> (-1.9779, -2.7717) centre (-2.4429, -3.4117) ccw
  line L58 (-1.6574, -3.505) -> (-1.7106, -3.9529)
  arc A100 (-1.7106, -3.9529) -> (-1.4527, -4.3593) centre (-1.3323, -3.9979) ccw
  arc A101 (-1.4527, -4.3593) -> (-1.387, -4.3807) centre (0, 0) ccw
  arc A102 (-1.387, -4.3807) -> (-0.9395, -4.2034) centre (-1.272, -4.0174) ccw
  line L59 (-0.9395, -4.2034) -> (-0.7193, -3.8098)
  circle A103 centre (0, 0) radius 1.5 projected
  point P0 (0, 0)
  dimension "d65" = 0.2
  constraints: 200 point on circle, 120 end point, 103 centre point, 2 coincident, 79 other
  measures "d65" radial gap between concentric circles of A25 A53
extrude "Extrusion13" cut sketch "Sketch9" against normal blind 1 contours L0 A1 A2 A3 L1 A4 L2 A5 L3 A6 A7 A8 L4 A9 L5 A10 L6 A11 A12 A13 L7 A14 L8 A15 L9 A16 A17 A18 L10 A19 L11 A20 L12 A21 A22 A23 L13 A24 L14 A25 L15 A26 A27 A28 L16 A29 L17 A30 L18 A31 A32 A33 L19 A34 L20 A35 L21 A36 A37 A38 L22 A39 L23 A40 L24 A41 A42 A43 L25 A44 L26 A45 L27 A46 A47 A48 L28 A49 L29 A50 | A53 L59 A102 A101 A100 L58 A99 L57 A98 L56 A97 A96 A95 L55 A94 L54 A93 L53 A92 A91 A90 L52 A89 L51 A88 L50 A87 A86 A85 L49 A84 L48 A83 L47 A82 A81 A80 L46 A79 L45 A78 L44 A77 A76 A75 L43 A74 L42 A73 L41 A72 A71 A70 L40 A69 L39 A68 L38 A67 A66 A65 L37 A64 L36 A63 L35 A62 A61 A60 L34 A59 L33 A58 L32 A57 A56 A55 L31 A54 L30 | A103
extrude "Extrusion15" add sketch "Sketch9" along normal blind 1 contours A0 | A51 | A52
chamfer "Chamfer5" distance 1.7 distance2 0.5 1 edges at (6.5, 0, -3.375) measured on face at (-2.9055, 4.0882, -3.375)
extrude "Extrusion14" add sketch "Sketch9" along normal blind 8.3 from surface at -1 separate body contours L0 A1 A2 A3 L1 A4 L2 A5 L3 A6 A7 A8 L4 A9 L5 A10 L6 A11 A12 A13 L7 A14 L8 A15 L9 A16 A17 A18 L10 A19 L11 A20 L12 A21 A22 A23 L13 A24 L14 A25 L15 A26 A27 A28 L16 A29 L17 A30 L18 A31 A32 A33 L19 A34 L20 A35 L21 A36 A37 A38 L22 A39 L23 A40 L24 A41 A42 A43 L25 A44 L26 A45 L27 A46 A47 A48 L28 A49 L29 A50
equation "\"da_pb\" = 2.5"
equation "\"da_fi\" = 25deg"
equation "\"da_hg\" = 0.75"
equation "\"da_bw\" = 1.05"
equation "\"da_rb\" = 0.2"
equation "\"da_rt\" = 0.3"
equation "\"da_a\" = 0.3"
equation "\"da_bf\" = 5.5"
equation "\"da_wf\" = 0.8"
equation "\"da_hf\" = 0.8"
